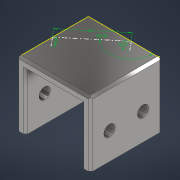
# Autodesk Inventor part: support_basePart_truss
Saved by Autodesk Inventor 2021 (Build 250183000, 183)
## iProperties
Created: 2021-05-24
Part Number: support_basePart_truss
Material: Steel, High Strength, Low Alloy
Document SubType Name: Modeling
Designer: Watchdog
Density: 7.85 g/cm^3
Appearance: Steel - Polished
Author: Watchdog
Autodesk Inventor part; units mm, degrees
ref_plane "YZ Plane" through (0, 0, 0) normal (1, 0, 0) x (0, 1, 0)
ref_plane "XZ Plane" through (0, 0, 0) normal (0, 1, 0) x (-1, 0, 0)
ref_plane "XY Plane" through (0, 0, 0) normal (0, 0, 1) x (1, 0, 0)
sketch "Sketch1" plane through (0, 0, 0) normal (0, 0, 1) x (1, 0, 0)
  line L0 (-33, 0) -> (33, 0)
  line L1 (33, 0) -> (33, -58)
  line L2 (33, -58) -> (-33, -58)
  line L3 (-33, -58) -> (-33, 0)
  point P0 (0, 0)
  dimension "d0" = 58
  dimension "d1" = 66
  dimension "d2" = 33
  dimension "d3" = 0
  constraints: 8 end point, 2 parallel, 1 horizontal, 1 perpendicular
  measures "d0" distance of L2.end L0.start
  measures "d1" distance of L0.start L0.end
  measures "d2" distance from line of point (0, 0) L3
  measures "d3" distance from line of point (0, 0) L0
extrude "clamp_base" add sketch "Sketch1" against normal blind 64
sketch "Sketch2" plane through (0, 0, 0) normal (0, 0, 1) x (1, 0, 0)
  line L0 (-25, -58) -> (25, -58)
  line L1 (25, -58) -> (25, -8)
  line L2 (25, -8) -> (-25, -8)
  line L3 (-25, -8) -> (-25, -58)
  line L4 (-33, -58) -> (33, -58) projected
  point P0 (0, 0)
  dimension "d6" = 50
  dimension "d7" = 50
  dimension "d8" = 25
  constraints: 8 end point, 2 parallel, 1 collinear, 1 horizontal, 1 perpendicular
  measures "d6" distance between parallel lines of L1 L3
  measures "d7" distance of L2.end L0.start
  measures "d8" distance from line of point (0, 0) L3
extrude "clamp_extrusion" cut sketch "Sketch2" against normal through all
sketch "Sketch4" plane through (-33, 0, 0) normal (0, 1, 0) x (1, 0, 0)
  line L0 (0, 64) -> (66, 64)
  line L1 (66, 64) -> (66, 0)
  line L2 (66, 0) -> (0, 0)
  line L3 (0, 0) -> (0, 64)
  line L4 (66, 0) -> (0, 0) projected
  line L5 (0, 64) -> (66, 64) projected
  line L6 (0, 0) -> (0, 64) projected
  line L7 (66, 0) -> (66, 64) projected
  point P0 (33, 0)
  dimension "d35" = 0
  dimension "d36" = 0
  dimension "d37" = 0
  dimension "d38" = 0
  constraints: 8 end point, 2 parallel, 1 horizontal, 1 perpendicular
  measures "d35" distance between parallel lines of L2 L4
  measures "d36" distance between parallel lines of L0 L5
  measures "d37" distance between parallel lines of L6 L3
  measures "d38" distance between parallel lines of L1 L7
extrude "platform" [suppressed]
sketch "Sketch8" plane through (33, -58, 0) normal (1, 0, 0) x (0, 0, -1)
  line L0 (0, 0) -> (0, 58) projected
  line L1 (64, 58) -> (64, 0) projected
  point P0 (17, 24.0271)
  point P1 (47, 24.0271)
  dimension "d51" = 17
  dimension "d60" = 30
  dimension "d61" = 64
  measures "d51" distance from line of L0 point (17, 24.027)
  measures "d60" distance of point (47, 24.027) point (17, 24.027)
  measures "d61" distance between parallel lines of L1 L0
hole "clampHole" at (33, -33.9729, -17) at (33, -33.9729, -47) direction (-1, 0, 0) diameter 10 end through all
fillet "Fillet1" [suppressed]
chamfer "Chamfer1" distance 2 angle 45 10 edges at (33, -29, -64) (33, -29, 0) (-33, -29, -64) (-33, -29, 0) (0, -8, -64) (25, -33, -64) (-25, -33, -64) (0, -8, 0) (-25, -33, 0) (25, -33, 0)
chamfer "Chamfer2" distance 2 angle 45 4 edges at (0, 0, -64) (33, 0, -32) (0, 0, 0) (-33, 0, -32)
sketch "Sketch11" plane through (-31, 0, -2) normal (0, 1, 0) x (1, 0, 0)
  line L0 (63, 61) -> (62, 60) projected
  line L1 (38.3022, 60) -> (0, 27.8606)
  line L2 (0, 0) -> (0, 60) projected
  line L3 (0, 60) -> (62, 60) projected
  line L4 (0, 27.8606) -> (6.4279, 20.2002)
  line L5 (38.3022, 60) -> (44.7301, 52.3396)
  dimension "d94" = 40
  dimension "d95" = 50
  dimension "d96" = 10
  dimension "d97" = 10
  constraints: 6 end point, 2 perpendicular, 2 point on line
  measures "d94" angle of L3 L1
  measures "d95" distance of L1.start L1.end
  measures "d96" distance of L1.end L4.end
  measures "d97" distance of L1.start L5.end
equation "\"d0\" = support_frame_squareBarDimension + support_baseClamp_thickness"
equation "\"d1\" = support_frame_squareBarDimension + 2 * support_baseClamp_thickness"
equation "\"d2\" = 0.5 * d1"
equation "\"d6\" = support_frame_squareBarDimension"
equation "\"d7\" = support_frame_squareBarDimension"
equation "\"d8\" = 0.5 * d6"
equation "\"d51\" = -0.5 * d60 + 0.5 * d61"
equation "\"d60\" = clampHoleSpacing"
equation "\"d13\" = support_baseClamp_platformThickness"
equation "\"d53\" = clampHoleDiameter"
equation "\"hoop_width_large\" = 51"
equation "\"buffer\" = 12"
equation "\"width\" = clampHoleDiameter + clampHoleSpacing + 2 * buffer"
equation "\"clampHoleSpacing\" = 30"
equation "\"clampHoleDiameter\" = support_frame_clampHoleDiameter"
equation "\"d12\" = -y + r - d15"
equation "\"d15\" = hoop_width_large"
equation "\"sleeveHoleDiameter\" = support_baseClamp_sleeveHoleDiameter"
equation "\"theta\" = hoop_angle_z"
equation "\"phi\" = support_baseClamp_sleeveSweepTerminationAngle"
equation "\"support_frame_squareBarDimension\" = 50"
equation "\"support_baseClamp_thickness\" = 8"
equation "\"support_baseClamp_sleeveHoleDiameter\" = 12"
equation "\"hoop_angle_z\" = 45deg"
equation "\"support_baseClamp_sleeveSweepTerminationAngle\" = 55deg"
equation "\"support_baseClamp_platformThickness\" = 15"
equation "\"support_baseClamp_platformWidthBuffer\" = 0"
equation "\"support_baseClamp_platformLengthBuffer\" = 35"
equation "\"rack_tooth_thickness\" = 5"
equation "\"rack_tooth_addendum\" = 5"
equation "\"rack_tooth_dedendum\" = 5"
equation "\"hoop_thickness_large\" = 4"
equation "\"hoop_width_medium\" = 33.7"
equation "\"hoop_thickness_medium\" = 3.2"
equation "\"hoop_width_small\" = 25.4"
equation "\"hoop_thickness_small\" = 2"
equation "\"hoop_bearing_length\" = 5deg"
equation "\"hoop_cable_diam\" = 5"
equation "\"hoop_cable_pulley_diam\" = 22"
equation "\"secure_arm_radii\" = 9"
equation "\"secure_arm_angle\" = 35deg"
equation "\"support_frame_endHoleBuffer\" = 45"
equation "\"hoop_tabs_thickness\" = 6"
equation "\"support_frame_squareBarThickness\" = 5"
equation "\"wheelchair_deployed_length\" = 1067"
equation "\"wheelchair_deployed_height\" = 914"
equation "\"hoop_tabs_hole\" = 12"
equation "\"wheelchair_deployed_width\" = 635"
equation "\"support_frame_squareBarFillet\" = 2"
equation "\"sm_varx_pinPlate_thickness\" = 5"
equation "\"sm_varx_member_tolerance\" = 0.5"
equation "\"sm_varx_pinPlate_holeDiameter\" = 5"
equation "\"sm_varx_squareBarThickness\" = 2.5"
equation "\"hoop_bushing23_radialInterference\" = 0"
equation "\"hoop_bushing12_radialInterference\" = 0"
equation "\"hoop_bushing12_od\" = 43"
equation "\"platformWidthExtension\" = 0"
equation "\"wheelchatir_pos_deploy_angle_0\" = 65deg"
equation "\"wheelchatir_pos_store_angle_0\" = 90deg"
equation "\"wheelchatir_pos_deploy_angle_1\" = 20deg"
equation "\"wheelchatir_pos_store_angle_1\" = 20deg"
equation "\"hoop_bushing23_od\" = 27.3"
equation "\"hoop_bushing12_thickness\" = 9.3"
equation "\"hoop_bushing23_thickness\" = 1.9"
equation "\"support_frame_clampHoleDiameter\" = 10"
equation "\"y\" = 450"
equation "\"r\" = 1650"
body "Solid1"
